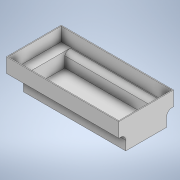
# Autodesk Inventor part: SamokatKorpus
Saved by Autodesk Inventor 2020.1 (Build 241239000, 239)
## iProperties
Created: 2023-01-15
Part Number: SamokatKorpus
Material: Типовые
Document SubType Name: Modeling
Designer: KirikDK
Density: 1 g/cm^3
Appearance: По умолчанию
Author: KirikDK
Autodesk Inventor part; units mm, degrees
ref_plane "YZ Plane" through (0, 0, 0) normal (1, 0, 0) x (0, 1, 0)
ref_plane "XZ Plane" through (0, 0, 0) normal (0, 1, 0) x (-1, 0, 0)
ref_plane "XY Plane" through (0, 0, 0) normal (0, 0, 1) x (1, 0, 0)
sketch "Эскиз1" plane through (0, 0, 0) normal (1, 0, 0) x (0, 1, 0)
  line L0 (19.3636, 71) -> (-32.2727, 71)
  line L1 (-32.2727, 71) -> (-32.2727, -71)
  line L2 (-32.2727, -71) -> (19.3636, -71)
  line L3 (19.3636, -71) -> (19.3636, 71)
  line L4 (67.7273, 95) -> (17.7273, 95)
  line L5 (17.7273, 95) -> (17.7273, -95)
  line L6 (17.7273, -95) -> (67.7273, -95)
  line L7 (67.7273, -95) -> (67.7273, 95)
  point P0 (0, 0)
  point P1 (17.7273, 71)
  point P2 (17.7273, -71)
  dimension "d0" = 142
  dimension "d1" = 190
  dimension "d2" = 50
  dimension "d3" = 24
  dimension "d4" = 24
  dimension "d5" = 50
  constraints: 16 end point, 4 parallel, 2 horizontal, 2 perpendicular
  measures "d0" distance of L2.end L0.start
  measures "d1" distance of L4.end L5.end
  measures "d2" distance between parallel lines of L1 L5
  measures "d3" distance from line of L4 L0.start
  measures "d4" distance from line of L6 L2.end
  measures "d5" distance of L4.start L4.end
extrude "Выдавливание1" add sketch "Эскиз1" along normal blind 355
fillet "Сопряжение1" radius 18 2 edges at (177.5, 17.7273, 71) (177.5, 17.7273, -71)
sketch "Эскиз2" plane through (0, 0, 0) normal (-1, 0, 0) x (0, 0, 1)
  line L0 (-95, 17.7273) -> (-95, 67.7273) projected
  line L1 (-95, 67.7273) -> (95, 67.7273)
  line L2 (95, 67.7273) -> (95, 17.7273)
  line L3 (95, 17.7273) -> (-95, 17.7273)
  line L4 (-95, 17.7273) -> (-95, 67.7273)
  line L5 (-71, -32.2727) -> (-71, -0.2727) projected
  line L6 (71, -32.2727) -> (-71, -32.2727) projected
  line L7 (71, -0.2727) -> (71, -32.2727) projected
  arc A0 (89, 17.7273) -> (71, -0.2727) centre (89, -0.2727) ccw projected
  line L8 (95, 17.7273) -> (89, 17.7273) projected
  line L9 (95, 67.7273) -> (95, 17.7273) projected
  line L10 (-95, 67.7273) -> (95, 67.7273) projected
  line L11 (-95, 17.7273) -> (-95, 67.7273) projected
  line L12 (-89, 17.7273) -> (-95, 17.7273) projected
  arc A1 (-71, -0.2727) -> (-89, 17.7273) centre (-89, -0.2727) ccw projected
  point P0 (0, 0)
  constraints: 8 end point, 2 parallel, 1 horizontal, 1 perpendicular
extrude "Выдавливание2" add sketch "Эскиз2" along normal blind 35 contours L0 L1 L2 L3
shell "Оболочка1" thickness 3 removed faces 1 at (95, 67.7273, -31.6667)
sketch "Эскиз3" plane through (352, -0.2727, 68) normal (0, 0, -1) x (-1, 0, 0)
  line L0 (349, 0) -> (0, 0) projected
  line L1 (0, 0) -> (0, -29) projected
  line L2 (349, -29) -> (0, -29) projected
  line L3 (349, 0) -> (349, -29) projected
  line L4 (349, 0) -> (0, 0) projected
  line L5 (349, 0) -> (0, 0)
  line L6 (0, 0) -> (0, 30)
  line L7 (0, 30) -> (349, 30)
  line L8 (349, 30) -> (349, 0)
  line L9 (0, 0) -> (349, 0) projected
  line L10 (349, -29) -> (349, 0) projected
  line L11 (349, -29) -> (0, -29) projected
  line L12 (0, -29) -> (0, 0) projected
  point P0 (352, 0.2727)
  constraints: 8 end point, 2 parallel, 1 horizontal, 1 perpendicular
sketch "Эскиз4" plane through (3, -0.2727, -68) normal (0, 0, 1) x (1, 0, 0)
  line L0 (349, 0) -> (0, 0) projected
  line L1 (0, -29) -> (0, 0) projected
  line L2 (0, -29) -> (349, -29) projected
  line L3 (349, -29) -> (349, 0) projected
  line L4 (0, 21) -> (0, 0) projected
  line L5 (349, 0) -> (0, 0)
  line L6 (0, 0) -> (0, 21)
  line L7 (0, 21) -> (349, 21)
  line L8 (349, 21) -> (349, 0)
  point P0 (-3, 0.2727)
  constraints: 8 end point, 2 parallel, 1 horizontal, 1 perpendicular
extrude "Выдавливание3" cut sketch "Эскиз3" against normal blind 1.5
extrude "Выдавливание4" cut sketch "Эскиз4" against normal blind 1.5
